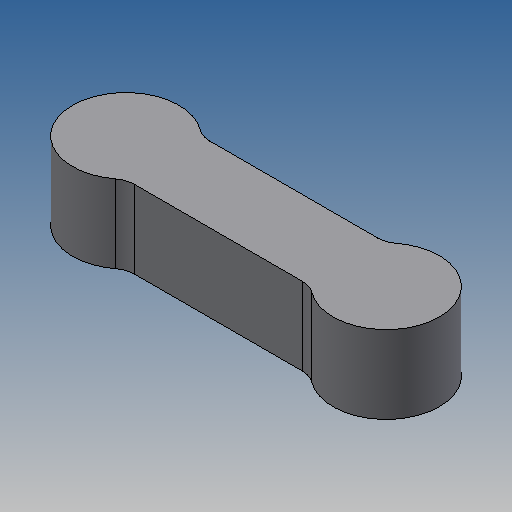
# Autodesk Inventor part: T2601_Conn
Saved by Autodesk Inventor 2025.3 (Build 293356000, 356)
## iProperties
Created: 2026-09-21
Part Number: T2601_Conn
Project: Nom Projet
Material: .
Description: Nom pièce
Document SubType Name: Modeling
Designer: jules
Authority: brut Ø
Mass: 0.000134406 g
Surface Area: 1.9014 cm^2
Volume: 0.134406 cm^3
Density: 0.001 g/cm^3
Appearance: Par défaut
Material number: ---
Author: jules
Autodesk Inventor part; units mm, degrees
ref_plane "Plan YZ" through (0, 0, 0) normal (1, 0, 0) x (0, 1, 0)
ref_plane "Plan XZ" through (0, 0, 0) normal (0, 1, 0) x (-1, 0, 0)
ref_plane "Plan XY" through (0, 0, 0) normal (0, 0, 1) x (1, 0, 0)
sketch "Esquisse1" plane through (0, 0, 0) normal (0, 0, 1) x (1, 0, 0)
  arc A0 (-3.575, 1.45) -> (-3.575, -1.45) centre (-5.025, 0) ccw
  line L0 (-5.025, 0) -> (-3.575, -1.45) construction
  line L1 (-5.025, 0) -> (-2.9744, 0) construction
  line L2 (-5.025, 0) -> (-3.575, 1.45) construction
  line L3 (-3.575, 1.45) -> (0, 1.45)
  line L4 (-3.575, -1.45) -> (0, -1.45)
  line L5 (0, -2.8709) -> (0, 2.8709) construction
  arc A1 (3.575, -1.45) -> (3.575, 1.45) centre (5.025, 0) ccw
  line L6 (3.575, 1.45) -> (0, 1.45)
  line L7 (3.575, -1.45) -> (0, -1.45)
  line L8 (-9.9059, 0) -> (9.9059, 0) construction
  point P0 (0, 0)
  dimension "d0" = 45
  dimension "d1" = 90
  dimension "d2" = 2.9
  dimension "d3" = 5.025
  constraints: 14 end point, 4 point on circle, 3 horizontal, 3 symmetric about line, 2 centre point, 1 collinear, 1 equal length, 1 other
  measures "d0" angle of L0 L1
  measures "d1" angle of L0 L2
  measures "d2" distance between parallel lines of L7 L6
  measures "d3" distance of L0.start point (0, 0)
extrude "Extrusion1" add sketch "Esquisse1" along normal blind 3
fillet "Congé1" radius 0.9 4 edges at (-3.575, -1.45, 1.5) (3.575, -1.45, 1.5) (3.575, 1.45, 1.5) (-3.575, 1.45, 1.5)
